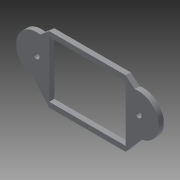
# Autodesk Inventor part: support_batteries
Saved by Autodesk Inventor 2014 SP1 (Build 180222100, 222)
## iProperties
Created: 2015-02-03
Part Number: support_batteries
Material: Générique
Document SubType Name: Modeling
Designer: astralien3000
Density: 1 g/cm^3
Appearance: Par défaut
Author: astralien3000
Autodesk Inventor part; units mm, degrees
note: some values were not read from the file. Chosen so that the rebuilt part matches the saved one: sketch regions of "Extrusion1".
ref_plane "YZ Plane" through (0, 0, 0) normal (1, 0, 0) x (0, 1, 0)
ref_plane "XZ Plane" through (0, 0, 0) normal (0, 1, 0) x (-1, 0, 0)
ref_plane "XY Plane" through (0, 0, 0) normal (0, 0, 1) x (1, 0, 0)
sketch "Esquisse1" plane through (0, 0, 0) normal (0, 1, 0) x (-1, 0, 0)
  line L0 (-37.5, 22) -> (37.5, 22)
  line L1 (37.5, 22) -> (37.5, -33)
  line L2 (37.5, -33) -> (-37.5, -33)
  line L3 (-37.5, -33) -> (-37.5, 22)
  line L4 (-37.5, 22) -> (37.5, 22)
  line L5 (37.5, 22) -> (37.5, 27)
  line L6 (37.5, 27) -> (-37.5, 27)
  line L7 (-37.5, 27) -> (-37.5, 22)
  line L8 (37.5, -33) -> (-37.5, -33)
  line L9 (-37.5, -33) -> (-37.5, -38)
  line L10 (-37.5, -38) -> (37.5, -38)
  line L11 (37.5, -38) -> (37.5, -33)
  circle A0 centre (-50, 0) radius 3
  arc A1 (-37.5, 15.6125) -> (-37.5, -15.6125) centre (-50, 0) ccw
  circle A2 centre (50, 0) radius 3
  arc A3 (37.5, -15.6125) -> (37.5, 15.6125) centre (50, 0) ccw
  line L12 (0, 0) -> (124.0045, 0) construction
  line L13 (-37.5, 27) -> (-70, 0)
  line L14 (-70, 0) -> (-37.5, -38)
  line L15 (37.5, 27) -> (70, 0)
  line L16 (37.5, -38) -> (70, 0)
  arc A4 (-37.5, -15.6125) -> (-37.5, 15.6125) centre (-50, 0) ccw
  arc A5 (30, 0) -> (37.5, -15.6125) centre (50, 0) ccw
  arc A6 (37.5, 15.6125) -> (30, 0) centre (50, 0) ccw
  dimension "d0" = 6
  dimension "d1" = 6
  dimension "d2" = 40
  dimension "d3" = 40
  dimension "d4" = 75
  dimension "d5" = 37.5
  dimension "d6" = 22
  dimension "d7" = 55
  dimension "d8" = 5
  dimension "d9" = 5
  dimension "d10" = 100
  dimension "d11" = 50
  constraints: 34 end point, 13 point on circle, 9 point on line, 7 centre point, 6 parallel, 4 perpendicular, 3 horizontal, 2 coincident, 2 collinear
  measures "d0" diameter of A2
  measures "d1" diameter of A0
  measures "d2" diameter of A1
  measures "d3" diameter of A3
  measures "d4" distance of L0.start L0.end
  measures "d5" distance from line of L3 L12.start
  measures "d6" distance from line of L12.start L0
  measures "d7" distance between parallel lines of L2 L0
  measures "d8" distance between parallel lines of L2 L10
  measures "d9" distance between parallel lines of L0 L6
  measures "d10" distance of A2.centre A0.centre
  measures "d11" distance of L12.start A1.centre
extrude "Extrusion1" add sketch "Esquisse1" along normal blind 5 contours L7 L6 L5 L0 | L3 A1 L13 L7 | L5 L15 A3 L1 | L3 A1 L14 L13 | A3 L15 L16 L1 | L3 L9 L14 A1 | L13 A1 | A3 L16 L11 L1 | A3 L15 | L2 L11 L10 L9 | A1 L14 | L16 A3
equation "\"d5\" = 0.5 * d4"
equation "\"d9\" = d8"
equation "\"d11\" = 0.5 * d10"
